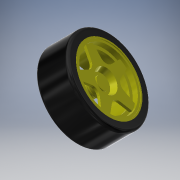
# Autodesk Inventor part: velg
Saved by Autodesk Inventor 2019 (Build 230136000, 136)
## iProperties
Created: 2017-01-19
Part Number: velg
Material: Generic
Document SubType Name: Modeling
Designer: schuer.davy
Density: 1 g/cm^3
Appearance: Default
Mass: 47.0024 g
Surface Area: 156.929 cm^2
Volume: 47.0024 cm^3
Author: schuer.davy
Autodesk Inventor part; units mm, degrees
ref_plane "YZ Plane" through (0, 0, 0) normal (1, 0, 0) x (0, 1, 0)
ref_plane "XZ Plane" through (0, 0, 0) normal (0, 1, 0) x (-1, 0, 0)
sketch "Sketch1" plane through (0, 0, 0) normal (0, 0, 1) x (1, 0, 0)
  line L0 (30.2, 0) -> (30.2, 5.65)
  line L1 (30.2, 5.65) -> (12, 5.65)
  arc A0 (12, 5.65) -> (10.15, 7.5) centre (10.15, 5.65) ccw
  line L2 (10.15, 7.5) -> (9, 7.5)
  line L3 (9, 7.5) -> (9, 8.5)
  line L4 (9, 8.5) -> (4.5, 10.5)
  line L5 (4.5, 10.5) -> (4.5, 20.5)
  line L6 (4.5, 20.5) -> (6.5, 20.5)
  line L7 (6.5, 20.5) -> (6.5, 23)
  line L8 (6.5, 23) -> (25.8, 23)
  line L9 (25.8, 23) -> (25.8, 26)
  line L10 (25.8, 26) -> (0, 26)
  line L11 (-6.04, 0) -> (36.24, 0) projected
  line L12 (0, 26) -> (0, 24.8)
  line L13 (0, 24.8) -> (0.5, 24.8)
  line L14 (2.5, 9) -> (6.5, 7.2222)
  line L15 (6.5, 7.2222) -> (6.5, 5)
  line L16 (6.5, 5) -> (5, 5)
  line L17 (5, 5) -> (5, 0)
  line L18 (0.5, 24.8) -> (0.5, 23)
  line L19 (0.5, 23) -> (2.5, 23)
  line L20 (2.5, 23) -> (2.5, 9)
  point P0 (0, 0)
  point P1 (21.1, 5.65)
  point P2 (0, 25.4)
  dimension "d2" = 11.3
  dimension "d3" = 52
  dimension "d4" = 15
  dimension "d5" = 3
  dimension "d6" = 7.5
  dimension "d7" = 25.8
  dimension "d8" = 21
  dimension "d9" = 1
  dimension "d10" = 18.2
  dimension "d11" = 3
  dimension "d12" = 1.2
  dimension "d13" = 0.5
  dimension "d14" = 10
  dimension "d15" = 1.5
  dimension "d16" = 5
  dimension "d17" = 30.2
  dimension "d18" = 18
  dimension "d19" = 2
  dimension "d20" = 41
  dimension "d23" = 2
  constraints: 40 end point, 11 perpendicular, 5 vertical, 3 parallel, 3 point on line, 2 midpoint, 2 point on circle, 1 centre point, 1 collinear, 1 horizontal alignment, 1 tangent, 1 vertical alignment
  measures "d2" diameter of L1 L11
  measures "d3" diameter of L10 L11
  measures "d4" diameter of L2 L11
  measures "d5" distance from line of L1.end L3
  measures "d6" distance from line of L5 L1.end
  measures "d7" distance of L9.end L10.end
  measures "d8" diameter of L4.end L11
  measures "d9" distance of L2.end L3.end
  measures "d10" distance of L0.end L1.end
  measures "d11" distance of L8.end L9.end
  measures "d12" distance of L10.end L12.end
  measures "d13" distance of L12.end L13.end
  measures "d14" diameter of L16 L11
  measures "d15" distance of L15.end L16.end
  measures "d16" distance between parallel lines of L12 L17
  measures "d17" distance from line of point (0, 0) L0
  measures "d18" diameter of L14.start L11
  measures "d19" distance of L5.end L6.end
  measures "d20" diameter of L6 L11
  measures "d23" distance of L18.end L19.end
revolve "Revolution1" add sketch "Sketch1" angle 360 about axis through (-10, 0, 0) along (1, 0, 0)
sketch "Sketch3" plane through (2.5, 0, 0) normal (-1, 0, 0) x (0, 0, 1)
  circle A0 centre (0, 0) radius 9 projected
  circle A1 centre (0, 0) radius 23 projected
  circle A2 centre (0, 0) radius 23 projected
  line L0 (3, -22.8035) -> (4.5531, -13.1907)
  arc A3 (10.9475, -8.6532) -> (4.5531, -13.1907) centre (9.9827, -14.068) ccw
  line L1 (10.9475, -8.6532) -> (20.534, -10.3613)
  circle A4 centre (0, 0) radius 5.65 construction
  line L2 (9.9827, -14.068) -> (0, 0) construction
  line L3 (0, -36.4) -> (0, 36.4) construction
  line L4 (22.6145, -4.1935) -> (13.9521, 0.2542)
  arc A5 (11.6127, 7.7377) -> (13.9521, 0.2542) centre (16.4643, 5.1469) ccw
  line L5 (16.4643, 5.1469) -> (0, 0) construction
  line L6 (11.6127, 7.7377) -> (16.1995, 16.3272)
  line L7 (10.9765, 20.2118) -> (4.0697, 13.3478)
  arc A6 (-3.7705, 13.4354) -> (4.0697, 13.3478) centre (0.1927, 17.2489) ccw
  line L8 (0.1927, 17.2489) -> (0, 0) construction
  line L9 (-3.7705, 13.4354) -> (-10.5221, 20.452)
  line L10 (-15.8306, 16.6851) -> (-11.4369, 7.9952)
  arc A7 (-13.9429, 0.5658) -> (-11.4369, 7.9952) centre (-16.3451, 5.5135) ccw
  line L11 (-16.3451, 5.5135) -> (0, 0) construction
  line L12 (-13.9429, 0.5658) -> (-22.7025, -3.6871)
  line L13 (-20.7604, -9.8998) -> (-11.1381, -8.4065)
  arc A8 (-4.8468, -13.0857) -> (-11.1381, -8.4065) centre (-10.2946, -13.8414) ccw
  line L14 (-10.2946, -13.8414) -> (0, 0) construction
  line L15 (-4.8468, -13.0857) -> (-3.5088, -22.7308)
  circle A9 centre (0, 0) radius 11.75 construction
  circle A10 centre (0, 0) radius 23 projected
  arc A11 (-15.8306, 16.6851) -> (-22.7025, -3.6871) centre (0, 0) ccw
  arc A12 (10.9765, 20.2118) -> (-10.5221, 20.452) centre (0, 0) ccw
  arc A13 (22.6145, -4.1935) -> (16.1995, 16.3272) centre (0, 0) ccw
  arc A14 (-20.7604, -9.8998) -> (-3.5088, -22.7308) centre (0, 0) ccw
  arc A15 (3, -22.8035) -> (20.534, -10.3613) centre (0, 0) ccw
  dimension "d24" = 3
  dimension "d25" = 21.5
  dimension "d28" = 360
  dimension "d30" = 23.5
  dimension "d31" = 5.5
  constraints: 30 end point, 24 point on circle, 11 centre point, 4 coincident, 3 tangent, 1 equal length, 51 other
  measures "d24" distance from line of L3 L0.start
  measures "d25" distance of L1.end L0.start
  measures "d30" diameter of A9
  measures "d31" radius of A8
extrude "Extrusion2" cut sketch "Sketch3" against normal blind 2 contours A1 L4 A5 L6 | L7 A6 L9 A1 | A1 L0 A3 L1 | L10 A7 L12 A1 | A1 L13 A8 L15
sketch "Sketch4" plane through (30.2, 0, 0) normal (1, 0, 0) x (0, 0, -1)
  line L0 (-1.825, 1.8519) -> (-1.825, -1.8519)
  line L1 (1.825, 1.8519) -> (1.825, -1.8519)
  arc A0 (-1.825, -1.8519) -> (1.825, -1.8519) centre (0, 0) ccw
  arc A1 (1.825, 1.8519) -> (-1.825, 1.8519) centre (0, 0) ccw
  dimension "d35" = 3.65
  dimension "d36" = 2.6
  constraints: 4 end point, 4 point on circle, 2 centre point, 2 parallel, 1 coincident, 1 concentric, 1 vertical
  measures "d35" distance between parallel lines of L1 L0
  measures "d36" radius of A1
extrude "Extrusion3" cut sketch "Sketch4" against normal blind 13
ref_plane "Work Plane1" through (0, 0, 0) normal (0, -1, 0) x (1, 0, 0)
sketch "Sketch5" plane through (0, 0, 0) normal (0, -1, 0) x (1, 0, 0)
  line L0 (25.8, -26) -> (25.8, 26) projected
  line L1 (0, -26) -> (0, 26) projected
  line L2 (0, 26) -> (25.8, 26) projected
  line L3 (23.8, 26) -> (2, 26)
  line L4 (2, 26) -> (2, 24)
  line L5 (2, 24) -> (23.8, 24)
  line L6 (23.8, 24) -> (23.8, 26)
  line L7 (-6.04, 0) -> (36.24, 0) projected
  point P0 (0, 0)
  dimension "d40" = 2
  dimension "d41" = 2
  dimension "d42" = 2
  constraints: 8 end point, 2 parallel, 1 horizontal, 1 perpendicular, 1 point on line
  measures "d40" distance between parallel lines of L0 L6
  measures "d41" distance between parallel lines of L1 L4
  measures "d42" distance between parallel lines of L2 L5
revolve "Revolution2" cut sketch "Sketch5" angle 360 about axis through (-10, 0, 0) along (1, 0, 0) contours L6 L5 L4 L2
sketch "Sketch6" plane through (0, 0, 0) normal (0, 0, 1) x (1, 0, 0)
  line L0 (2, 24) -> (23.8, 24) projected
  line L1 (23.8, -26) -> (23.8, 26) projected
  line L2 (23.8, 26) -> (25.8, 26) projected
  line L3 (2, 26) -> (2, -26) projected
  line L4 (0, 26) -> (2, 26) projected
  arc A0 (2.6, 32.5) -> (0.1, 30) centre (2.6, 30) ccw
  line L5 (2.6, 32.5) -> (23.2, 32.5)
  arc A1 (25.7, 30) -> (23.2, 32.5) centre (23.2, 30) ccw
  line L6 (-6.6357, 0) -> (36.3393, 0) projected
  line L7 (0.1, 30) -> (0.1, 26)
  line L8 (25.7, 30) -> (25.7, 26)
  point P0 (0, 0)
  dimension "d44" = 65
  dimension "d45" = 2.5
  dimension "d46" = 0.1
  dimension "d47" = 0.1
  constraints: 6 end point, 4 point on circle, 4 tangent, 2 centre point, 2 point on line, 2 vertical, 1 equal radius
  measures "d44" diameter of L5 L6
  measures "d45" radius of A0
  measures "d46" distance of L4.start L7.end
  measures "d47" distance of L2.end L8.end
revolve "Revolution3" add sketch "Sketch6" angle 360 about axis through (-10, 0, 0) along (1, 0, 0) contours L3 L4 L7 A0 L5 A1 L8 L2 L1 L0
scale "Scale1" factors (0.9, 0.9, 0.9) then translate (1.29, 0, 0) bodies 1
equation "\"d41\" = d40"
body "Solid1"
